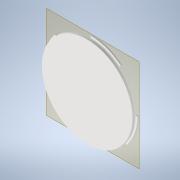
# Autodesk Inventor part: GehaeuseteilA
Saved by Autodesk Inventor 2020.2 (Build 242310000, 310)
## iProperties
Created: 2020-02-12
Part Number: GehaeuseteilA
Material: Generisch
Document SubType Name: Modeling
Designer: Max
Density: 1 g/cm^3
Appearance: Vorgabe
Author: Max
Autodesk Inventor part; units mm, degrees
ref_plane "YZ Plane" through (0, 0, 0) normal (1, 0, 0) x (0, 1, 0)
ref_plane "XZ Plane" through (0, 0, 0) normal (0, 1, 0) x (-1, 0, 0)
sketch "Skizze2" plane through (0, 0, 0) normal (0, 0, 1) x (1, 0, 0)
  circle A0 centre (0, 0) radius 64.5
  point P0 (1.5625, 1.8697)
  dimension "d1" = 129
  constraints: 1 centre point, 1 coincident, 1 other
  measures "d1" diameter of A0
extrude "Extrusion1" add sketch "Skizze2" along normal blind 3
ref_plane "Arbeitsebene1" through (0, 0, -5) normal (0, 0, 1) x (1, 0, 0)
sketch "Skizze16" plane through (0, 0, 0) normal (0, 0, -1) x (-1, 0, 0)
  circle A0 centre (0, 0) radius 58.3
  circle A1 centre (0, 0) radius 64.5 projected
  circle A2 centre (0, 0) radius 56.3
  dimension "d49" = 6.2
  dimension "d50" = 2
  constraints: 2 centre point, 2 coincident
  measures "d49" radial gap between concentric circles of A1 A0
  measures "d50" radial gap between concentric circles of A0 A2
extrude "Extrusion2" add sketch "Skizze16" along normal blind 4.1 contours A0
sketch "Skizze17" plane through (0, 0, -4.1) normal (0, 0, -1) x (-1, 0, 0)
  circle A0 centre (0, 0) radius 63.8
  circle A1 centre (0, 0) radius 66.5
  circle A2 centre (0, 0) radius 58.3 projected
  dimension "d53" = 2.7
  dimension "d54" = 127.6
  constraints: 2 centre point, 2 coincident, 1 concentric
  measures "d53" radial gap between concentric circles of A0 A1
  measures "d54" diameter of A0
extrude "Extrusion3" add sketch "Skizze17" against normal blind 2 contours A1
sketch "Skizze18" plane through (0, 0, 0) normal (0, 0, -1) x (-1, 0, 0)
  circle A0 centre (0, 0) radius 66.5 projected
  line L0 (0, 0) -> (0, 66.5)
  line L1 (0, 0) -> (50.942, 42.7454)
  line L2 (0, 0) -> (66.5, 0)
  line L3 (0, 0) -> (42.096, -50.168)
  line L4 (0, 0) -> (0, -65.4897)
  line L5 (0, 0) -> (-50.942, -42.7454)
  line L6 (0, 0) -> (-66.5, 0)
  line L7 (0, 0) -> (-42.7454, 50.942)
  arc A1 (66.5, 0) -> (50.942, 42.7454) centre (0, 0) ccw
  arc A2 (0, 66.5) -> (-42.7454, 50.942) centre (0, 0) ccw
  arc A3 (-66.5, 0) -> (-50.942, -42.7454) centre (0, 0) ccw
  arc A4 (0, -65.4897) -> (42.096, -50.168) centre (4.6329, -12.7289) ccw
  point P0 (-50.942, -42.7454)
  point P1 (-11.5476, -65.4897)
  point P2 (42.7454, -50.942)
  point P3 (20.6268, -63.2201)
  point P4 (24.8361, -61.6881)
  dimension "d57" = 50
  dimension "d58" = 50
  dimension "d59" = 50
  dimension "d60" = 40
  dimension "d61" = 50
  dimension "d64" = 40
  constraints: 16 end point, 10 point on circle, 4 centre point, 2 coincident, 1 horizontal, 1 perpendicular, 1 point on line, 1 vertical
  measures "d57" angle of L1 L0
  measures "d58" angle of L2 L3
  measures "d59" angle of L4 L5
  measures "d60" angle of L3 L4
  measures "d61" angle of L6 L7
  measures "d64" angle of L1 L2
extrude "Extrusion4" cut sketch "Skizze18" along normal up to surface (4.1 mm away) contours A0 A4 L3 L2 | L1 L0 A0 | L4 A4 A0 L5 | L6 A0 L7
